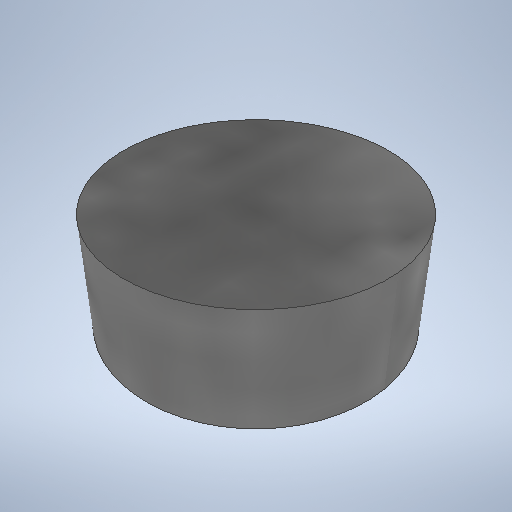
# Autodesk Inventor part: Motor
Saved by Autodesk Inventor 2025.2 (Build 292293000, 293)
## iProperties
Created: 2026-02-20
Part Number: Motor
Material: 一般
Document SubType Name: Modeling
Designer: naka6
Density: 1 g/cm^3
Appearance: 鋼材 メッキ
Author: naka6
Autodesk Inventor part; units mm, degrees
ref_plane "YZ Plane" through (0, 0, 0) normal (1, 0, 0) x (0, 1, 0)
ref_plane "XZ Plane" through (0, 0, 0) normal (0, 1, 0) x (-1, 0, 0)
ref_plane "XY Plane" through (0, 0, 0) normal (0, 0, 1) x (1, 0, 0)
sketch "スケッチ1" plane through (0, 0, 0) normal (0, 1, 0) x (-1, 0, 0)
  circle A0 centre (0, 0) radius 5
  dimension "d0" = 10
  constraints: 1 centre point, 1 coincident
  measures "d0" diameter of A0
extrude "押し出し1" add sketch "スケッチ1" along normal blind 4
